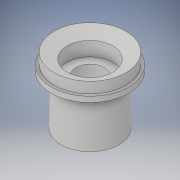
# Autodesk Inventor part: Phenlic
Saved by Autodesk Inventor 2017 (Build 210142000, 142)
## iProperties
Created: 2016-07-19
Part Number: Phenlic
Material: Generic
Document SubType Name: Modeling
Designer: Bill
Density: 1 g/cm^3
Appearance: Default
Author: Bill
Autodesk Inventor part; units mm, degrees
ref_plane "YZ Plane" through (0, 0, 0) normal (1, 0, 0) x (0, 1, 0)
ref_plane "XZ Plane" through (0, 0, 0) normal (0, 1, 0) x (-1, 0, 0)
ref_plane "XY Plane" through (0, 0, 0) normal (0, 0, 1) x (1, 0, 0)
sketch "Sketch1" plane through (0, 0, 0) normal (0, 0, 1) x (1, 0, 0)
  line L0 (-67.183, -7.8688) -> (-65.1298, 106.4127)
  line L1 (-67.183, -7.8688) -> (-60.833, -7.8688)
  line L2 (-65.1298, 106.4127) -> (-89.4122, 106.4127)
  line L3 (-89.4122, 106.4127) -> (-89.4122, 119.1127)
  line L4 (-89.4122, 119.1127) -> (-83.0622, 119.1127)
  line L5 (-83.0622, 119.1127) -> (-83.0622, 144.5127)
  line L6 (-83.0622, 144.5127) -> (-32.4858, 144.5127) construction
  line L7 (-60.833, -7.8688) -> (-32.6241, 97.4082)
  line L8 (-32.6241, 97.4082) -> (-52.858, 97.4082)
  line L9 (-52.858, 97.4082) -> (-52.858, 130.4282)
  line L10 (-83.0622, 144.5127) -> (-52.858, 130.4282)
  line L11 (0, -38.3452) -> (0, 174.989) projected
  point P0 (0, 0)
  dimension "d0" = 6.35
  dimension "d1" = 60.833
  dimension "d2" = 114.3
  dimension "d4" = 12.7
  dimension "d5" = 24.2824
  dimension "d6" = 25.4
  dimension "d9" = 6.35
  dimension "d10" = 105
  dimension "d11" = 25
  dimension "d13" = 33.02
  constraints: 22 end point, 5 horizontal, 2 perpendicular
  measures "d0" distance of L0.start L1.end
  measures "d1" horizontal distance of point (0, 0) L1.end
  measures "d2" distance of L0.start L0.end
  measures "d4" distance of L2.end L3.end
  measures "d5" distance of L0.end L2.end
  measures "d6" distance of L4.end L5.end
  measures "d9" distance of L3.end L4.end
  measures "d10" angle of L1 L7
  measures "d11" angle of L6 L10
  measures "d13" distance of L8.end L9.end
revolve "Revolution1" add sketch "Sketch1" angle 360 about axis through (0, -10, 0) along (0, 1, 0)
body "Solid1"
